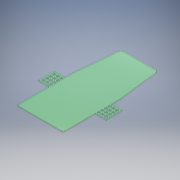
# Autodesk Inventor part: Base
Saved by Autodesk Inventor 2017 (Build 210142000, 142)
## iProperties
Created: 2017-04-01
Part Number: Base
Material: Acrylic
Document SubType Name: Modeling
Designer: Nick
Density: 1.188 g/cm^3
Appearance: Transparent - Clear
Author: Nick
Autodesk Inventor part; units mm, degrees
ref_plane "YZ Plane" through (0, 0, 0) normal (1, 0, 0) x (0, 1, 0)
ref_plane "XZ Plane" through (0, 0, 0) normal (0, 1, 0) x (-1, 0, 0)
ref_plane "XY Plane" through (0, 0, 0) normal (0, 0, 1) x (1, 0, 0)
sketch "Sketch1" plane through (0, 0, 0) normal (0, 0, 1) x (1, 0, 0)
  line L0 (-150, 243.8158) -> (150, 243.8158) construction
  line L1 (150, 243.8158) -> (150, -220) construction
  line L2 (150, -220) -> (-150, -220) construction
  line L3 (-150, -220) -> (-150, 243.8158) construction
  line L4 (0, 0) -> (220, 0)
  line L5 (-60, -122.4751) -> (60, -122.4751)
  line L6 (65, -117.4751) -> (65, -32.4751)
  line L7 (65, -32.4751) -> (95, -32.4751)
  line L8 (95, -32.4751) -> (95, 12.5249)
  line L9 (95, 12.5249) -> (65, 12.5249)
  line L10 (65, 12.5249) -> (65, 36.9333)
  line L11 (45.5834, 157.5249) -> (-48.2334, 157.5249)
  line L12 (-53.2078, 153.0301) -> (-65, 36.9333)
  line L13 (-65, 12.5249) -> (-95, 12.5249)
  line L14 (-95, 12.5249) -> (-95, -32.4751)
  line L15 (-95, -32.4751) -> (-65, -32.4751)
  line L16 (-65, -32.4751) -> (-65, -117.4751)
  line L17 (-90, 7.5249) -> (-85, 7.5249)
  line L18 (-85, 7.5249) -> (-85, 2.5249)
  line L19 (-85, 2.5249) -> (-90, 2.5249)
  line L20 (-90, 2.5249) -> (-90, 7.5249)
  line L21 (-90, -7.4751) -> (-90, -2.4751)
  line L22 (-90, -2.4751) -> (-85, -2.4751)
  line L23 (-85, -2.4751) -> (-85, -7.4751)
  line L24 (-85, -7.4751) -> (-90, -7.4751)
  line L25 (-90, -17.4751) -> (-90, -12.4751)
  line L26 (-90, -12.4751) -> (-85, -12.4751)
  line L27 (-85, -12.4751) -> (-85, -17.4751)
  line L28 (-85, -17.4751) -> (-90, -17.4751)
  line L29 (-90, -27.4751) -> (-90, -22.4751)
  line L30 (-90, -22.4751) -> (-85, -22.4751)
  line L31 (-85, -22.4751) -> (-85, -27.4751)
  line L32 (-85, -27.4751) -> (-90, -27.4751)
  line L33 (-80, 2.5249) -> (-80, 7.5249)
  line L34 (-80, 7.5249) -> (-75, 7.5249)
  line L35 (-75, 7.5249) -> (-75, 2.5249)
  line L36 (-75, 2.5249) -> (-80, 2.5249)
  line L37 (-80, -7.4751) -> (-80, -2.4751)
  line L38 (-80, -2.4751) -> (-75, -2.4751)
  line L39 (-75, -2.4751) -> (-75, -7.4751)
  line L40 (-75, -7.4751) -> (-80, -7.4751)
  line L41 (-80, -17.4751) -> (-80, -12.4751)
  line L42 (-80, -12.4751) -> (-75, -12.4751)
  line L43 (-75, -12.4751) -> (-75, -17.4751)
  line L44 (-75, -17.4751) -> (-80, -17.4751)
  line L45 (-80, -27.4751) -> (-80, -22.4751)
  line L46 (-80, -22.4751) -> (-75, -22.4751)
  line L47 (-75, -22.4751) -> (-75, -27.4751)
  line L48 (-75, -27.4751) -> (-80, -27.4751)
  line L49 (-70, 2.5249) -> (-70, 7.5249)
  line L50 (-70, 7.5249) -> (-65, 7.5249)
  line L51 (-65, 7.5249) -> (-65, 2.5249)
  line L52 (-65, 2.5249) -> (-70, 2.5249)
  line L53 (-70, -7.4751) -> (-70, -2.4751)
  line L54 (-70, -2.4751) -> (-65, -2.4751)
  line L55 (-65, -2.4751) -> (-65, -7.4751)
  line L56 (-65, -7.4751) -> (-70, -7.4751)
  line L57 (-70, -17.4751) -> (-70, -12.4751)
  line L58 (-70, -12.4751) -> (-65, -12.4751)
  line L59 (-65, -12.4751) -> (-65, -17.4751)
  line L60 (-65, -17.4751) -> (-70, -17.4751)
  line L61 (-70, -27.4751) -> (-70, -22.4751)
  line L62 (-70, -22.4751) -> (-65, -22.4751)
  line L63 (-65, -22.4751) -> (-65, -27.4751)
  line L64 (-65, -27.4751) -> (-70, -27.4751)
  line L65 (0, -285.0452) -> (0, 260.9735) construction
  line L66 (90, 7.5249) -> (85, 7.5249)
  line L67 (85, 7.5249) -> (85, 2.5249)
  line L68 (85, 2.5249) -> (90, 2.5249)
  line L69 (90, 2.5249) -> (90, 7.5249)
  line L70 (90, -7.4751) -> (90, -2.4751)
  line L71 (90, -2.4751) -> (85, -2.4751)
  line L72 (85, -2.4751) -> (85, -7.4751)
  line L73 (85, -7.4751) -> (90, -7.4751)
  line L74 (90, -17.4751) -> (90, -12.4751)
  line L75 (90, -12.4751) -> (85, -12.4751)
  line L76 (85, -12.4751) -> (85, -17.4751)
  line L77 (85, -17.4751) -> (90, -17.4751)
  line L78 (90, -27.4751) -> (90, -22.4751)
  line L79 (90, -22.4751) -> (85, -22.4751)
  line L80 (85, -22.4751) -> (85, -27.4751)
  line L81 (85, -27.4751) -> (90, -27.4751)
  line L82 (80, 2.5249) -> (80, 7.5249)
  line L83 (80, 7.5249) -> (75, 7.5249)
  line L84 (75, 7.5249) -> (75, 2.5249)
  line L85 (75, 2.5249) -> (80, 2.5249)
  line L86 (80, -7.4751) -> (80, -2.4751)
  line L87 (80, -2.4751) -> (75, -2.4751)
  line L88 (75, -2.4751) -> (75, -7.4751)
  line L89 (75, -7.4751) -> (80, -7.4751)
  line L90 (80, -17.4751) -> (80, -12.4751)
  line L91 (80, -12.4751) -> (75, -12.4751)
  line L92 (75, -12.4751) -> (75, -17.4751)
  line L93 (75, -17.4751) -> (80, -17.4751)
  line L94 (80, -27.4751) -> (80, -22.4751)
  line L95 (80, -22.4751) -> (75, -22.4751)
  line L96 (75, -22.4751) -> (75, -27.4751)
  line L97 (75, -27.4751) -> (80, -27.4751)
  line L98 (70, 2.5249) -> (70, 7.5249)
  line L99 (70, 7.5249) -> (65, 7.5249)
  line L100 (65, 7.5249) -> (65, 2.5249)
  line L101 (65, 2.5249) -> (70, 2.5249)
  line L102 (70, -7.4751) -> (70, -2.4751)
  line L103 (70, -2.4751) -> (65, -2.4751)
  line L104 (65, -2.4751) -> (65, -7.4751)
  line L105 (65, -7.4751) -> (70, -7.4751)
  line L106 (70, -17.4751) -> (70, -12.4751)
  line L107 (70, -12.4751) -> (65, -12.4751)
  line L108 (65, -12.4751) -> (65, -17.4751)
  line L109 (65, -17.4751) -> (70, -17.4751)
  line L110 (70, -27.4751) -> (70, -22.4751)
  line L111 (70, -22.4751) -> (65, -22.4751)
  line L112 (65, -22.4751) -> (65, -27.4751)
  line L113 (65, -27.4751) -> (70, -27.4751)
  line L114 (-65, 36.9333) -> (-65, 12.5249)
  line L115 (65, 36.9333) -> (50.5452, 153.142)
  arc A0 (-48.2334, 157.5249) -> (-53.2078, 153.0301) centre (-48.2334, 152.5249) ccw
  arc A1 (50.5452, 153.142) -> (45.5834, 157.5249) centre (45.5834, 152.5249) ccw
  arc A2 (-65, -117.4751) -> (-60, -122.4751) centre (-60, -117.4751) ccw
  arc A3 (60, -122.4751) -> (65, -117.4751) centre (60, -117.4751) ccw
  point P0 (-65, -122.4751)
  point P1 (65, -122.4751)
  point P2 (50, 157.5249)
  point P3 (-52.7512, 157.5249)
  dimension "d3" = 220
  dimension "d6" = 150
  dimension "d7" = 300
  dimension "d8" = 220
  dimension "d10" = 130
  dimension "d11" = 65
  dimension "d14" = 30
  dimension "d15" = 30
  dimension "d16" = 45
  dimension "d18" = 122.4751
  dimension "d19" = 280
  dimension "d20" = 90
  dimension "d21" = 30
  dimension "d22" = 5
  dimension "d23" = 5
  dimension "d24" = 5
  dimension "d25" = 5
  dimension "d32" = 463.8158
  dimension "d35" = 10
  dimension "d38" = 10
  dimension "d43" = 5
  dimension "d52" = 24.4085
  dimension "d60" = 5
  dimension "d61" = 5
  constraints: 225 end point, 48 symmetric about line, 13 point on line, 8 point on circle, 8 tangent, 6 perpendicular, 4 centre point, 4 horizontal, 3 parallel, 3 vertical, 2 equal radius, 2 vertical alignment, 1 horizontal alignment, 90 other
  measures "d3" distance of L4.start L4.end
  measures "d6" horizontal distance of L4.start L2.end
  measures "d7" distance between parallel lines of L1 L3
  measures "d8" vertical distance of L2.end L4.start
  measures "d10" distance of point (-65, -122.475) point (65, -122.475)
  measures "d11" horizontal distance of point (-65, -122.475) L4.start
  measures "d14" distance of L6.end L7.end
  measures "d15" distance of L14.end L15.end
  measures "d16" distance of L7.end L8.end
  measures "d18" distance from line of L5 L4.start
  measures "d19" distance between parallel lines of L5 L11
  measures "d20" distance of point (65, -122.475) L6.end
  measures "d21" distance of L13.start L13.end
  measures "d22" distance between parallel lines of L20 L14
  measures "d23" distance of L19.end L17.start
  measures "d24" distance of L17.start L17.end
  measures "d25" distance between parallel lines of L13 L17
  measures "d32" distance between parallel lines of L2 L0
  measures "d35" distance of L19.end L21.start
  measures "d38" distance of L19.end L33.start
  measures "d43" distance between parallel lines of L8 L69
  measures "d52" distance of L12.end L13.start
  measures "d60" radius of A0
  measures "d61" radius of A1
extrude "Extrusion1" add sketch "Sketch1" along normal blind 3
equation "\"d6\" = 0.5 * d7"
equation "\"d11\" = 0.5 * d10"
equation "\"d15\" = d14"
equation "\"d21\" = d15"
body "Solid1"
